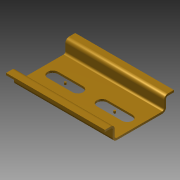
# Autodesk Inventor part: D0032871-0
Saved by Autodesk Inventor 2016 (Build 200138000, 138)
## iProperties
CDBZ_nummer: D0032871
CDBZ_index: 0
Category: IPart-Factory
Shininess: 27.0
Length Units: 11269
Angle Units: 11279
Time Units: 11290
Mass Units: 11283
Length Display Precision: 3
Angle Display Precision: 2
Created: 2001-08-16
Material: S235JR (gelbverzinkt)
Document SubType Name: Blech
Description: Tragschiene
User Status: Freigegeben
Mass: 16.4383 g
Surface Area: 44.6937 cm^2
Volume: 2.09405 cm^3
Density: 7.85 g/cm^3
Sheet Metal Rule: Default
Appearance: Metal-Brass
Density: 0.0
Volumn: 0.0
Area: 0.0
PropertySet Name: Model Information
Control State: 0
Master: False
Checked Out: False
Länge: 200,000 mm
Revision Number: 1
Autodesk Inventor part; units mm, degrees
ref_plane "YZ Ebene" through (0, 0, 0) normal (1, 0, 0) x (0, 1, 0)
ref_plane "XZ Ebene" through (0, 0, 0) normal (0, 1, 0) x (-1, 0, 0)
ref_plane "XY Ebene" through (0, 0, 0) normal (0, 0, 1) x (1, 0, 0)
sketch "Skizze1" plane through (0, 0, 0) normal (0, 0, 1) x (1, 0, 0)
  line L0 (0, -12.5) -> (200, -12.5)
  line L1 (200, -12.5) -> (200, 12.5)
  line L2 (200, 12.5) -> (0, 12.5)
  line L3 (0, 12.5) -> (0, -12.5)
  line L4 (6.15, 2.65) -> (18.85, 2.65)
  arc A0 (18.85, -2.65) -> (18.85, 2.65) centre (18.85, 0) ccw
  line L5 (18.85, -2.65) -> (6.15, -2.65)
  arc A1 (6.15, 2.65) -> (6.15, -2.65) centre (6.15, 0) ccw
  circle A2 centre (12.5, 0) radius 0.5
  point P0 (0, 0)
  dimension "Länge" = 200
  dimension "breite" = 25
  dimension "d2" = 2.65
  dimension "d4" = 12.7
  dimension "mitte" = 12.5
  dimension "d22" = 6.15
  dimension "d43" = 6.35
  dimension "d44" = 1
  dimension "d45" = 12.5
  constraints: 12 end point, 4 point on circle, 4 tangent, 3 centre point, 3 parallel, 2 horizontal alignment, 2 perpendicular, 1 horizontal, 1 vertical alignment, 1 other
  measures "Länge" distance of L0.start L0.end
  measures "breite" distance of L2.end L0.start
  measures "d2" radius of A1
  measures "d4" distance of L4.start L4.end
  measures "mitte" vertical distance of A1.centre L0.start
  measures "d22" horizontal distance of A1.centre L0.start
  measures "d43" distance of A2.centre A1.centre
  measures "d44" diameter of A2
  measures "d45" distance from line of point (0, 0) L0
extrude "Platte1" add sketch "Skizze1" along normal blind 1 contours L3 L2 L1 L0 | L4 A0 L5 A1 | A2
sketch "Skizze3" plane through (0, -12.5, 0) normal (0, 1, 0) x (-1, 0, 0)
  line L0 (0, 0) -> (-200, 0)
  line L1 (-200, 0) -> (-200, 6.5)
  line L2 (-200, 6.5) -> (0, 6.5)
  line L3 (0, 6.5) -> (0, 0)
  constraints: 6 end point, 1 horizontal, 1 perpendicular, 1 vertical
sheet face with bend "Lasche1" sketch "Skizze3" thickness 1 toward (0, -1, 0) bend radius 1 relief straight relief width 1 relief depth 0.5
bend "Biegung1"
sketch "Skizze4" plane through (200, 12.5, 0) normal (0, -1, 0) x (1, 0, 0)
  line L0 (0, 0) -> (-200, 0)
  line L1 (-200, 0) -> (-200, 6.5)
  line L2 (-200, 6.5) -> (0, 6.5)
  line L3 (0, 6.5) -> (0, 0)
  constraints: 6 end point, 1 horizontal, 1 perpendicular, 1 vertical
sheet face with bend "Lasche2" sketch "Skizze4" thickness 1 toward (0, 1, 0) bend radius 1 relief straight relief width 1 relief depth 0.5
bend "Biegung2"
sketch "Skizze5" plane through (0, 12.5, 6.5) normal (0, 0, -1) x (-1, 0, 0)
  line L0 (0, 0) -> (-200, 0)
  line L1 (-200, 0) -> (-200, 5)
  line L2 (-200, 5) -> (0, 5)
  line L3 (0, 5) -> (0, 0)
  constraints: 6 end point, 1 horizontal, 1 perpendicular, 1 vertical
sheet face with bend "Lasche3" sketch "Skizze5" thickness 1 toward (0, 0, 1) bend radius 1 relief straight relief width 1 relief depth 0.5
bend "Biegung3"
sketch "Skizze6" plane through (200, -12.5, 6.5) normal (0, 0, -1) x (-1, 0, 0)
  line L0 (0, 0) -> (200, 0)
  line L1 (200, 0) -> (200, -5)
  line L2 (200, -5) -> (0, -5)
  line L3 (0, -5) -> (0, 0)
  constraints: 6 end point, 1 horizontal, 1 perpendicular, 1 vertical
sheet face with bend "Lasche4" sketch "Skizze6" thickness 1 toward (0, 0, 1) bend radius 1 relief straight relief width 1 relief depth 0.5
bend "Biegung4"
extrude "Extrusion1" cut sketch "Skizze1" along normal through all contours L4 A0 L5 A1
pattern_linear "Rechteckige Anordnung1" count 9 spacing 25 along (1, 0, 0) of "Extrusion1"
equation "\"mitte\" = 0.5 * breite"
equation "\"d43\" = 0.5 * d4"
equation "\"d45\" = 0.5 * breite"
equation "\"d11\" = Biegeradius"
equation "\"d29\" = BreiteBiegungsfreistellung"
equation "\"d31\" = MinimalRest"
equation "\"d30\" = TiefeBiegungsfreistellung"
equation "\"d41\" = Biegeradius"
equation "\"d14\" = Biegeradius"
equation "\"d32\" = BreiteBiegungsfreistellung"
equation "\"d34\" = MinimalRest"
equation "\"d33\" = TiefeBiegungsfreistellung"
equation "\"d42\" = Biegeradius"
equation "\"d17\" = Biegeradius"
equation "\"MinimalRest\" = 2 * Objekthöhe"
equation "\"BreiteBiegungsfreistellung\" = Objekthöhe"
equation "\"d35\" = BreiteBiegungsfreistellung"
equation "\"d36\" = TiefeBiegungsfreistellung"
equation "\"d37\" = MinimalRest"
equation "\"d20\" = Biegeradius"
equation "\"d38\" = BreiteBiegungsfreistellung"
equation "\"d39\" = TiefeBiegungsfreistellung"
equation "\"d40\" = MinimalRest"
equation "\"Biegeradius\" = Objekthöhe"
equation "\"TiefeBiegungsfreistellung\" = 0.5 * Objekthöhe"
equation "\"GrößeEckenfreistellung\" = 4 * Objekthöhe"
equation "\"d8\" = Biegeradius"
equation "\"Übergangsradius\" = Biegeradius"
equation "\"JacobiRadiusGröße\" = Objekthöhe"
equation "\"Abstandsgröße\" = Objekthöhe"
equation "\"Objekthöhe\" = 1"
body "Solid1"
